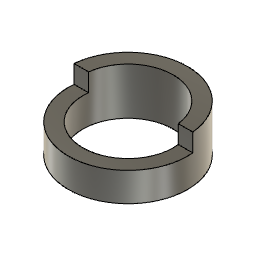
DISP_Ring_V2 v1 (Autodesk Fusion 360 design; units mm, degrees)
Autodesk Fusion 360 part; units mm, degrees
note: some values were not read from the file. Set by a fixed rule: which sketch regions a step uses.
sketch "Sketch1" plane through (0, 0, 0) normal (0, 0, 1) x (1, 0, 0)
  circle A0 centre (0, 0) radius 16.5
  circle A1 centre (0, 0) radius 12.5
  dimension "d1" = 33
  dimension "d2" = 25
  constraint coincident A0.centre A1.centre
  measures "d1" diameter of A0
  measures "d2" diameter of A1
extrude "Extrude1" add sketch "Sketch1" along normal blind 8
sketch "Sketch2" plane through (0, 0, 8) normal (0, 0, 1) x (-1, 0, 0)
  circle A0 centre (0, 0) radius 12.5
  circle A1 centre (0, 0) radius 16.5
  line L0 (-0.0363, -16.5) -> (-0.0363, -1.5) construction
  line L1 (-0.0363, -1.5) -> (16.4317, -1.5) construction
  line L2 (16.4317, -1.5) -> (-16.4317, -1.5)
  line L3 (-16.4317, -1.5) -> (-13.3757, -8.3419)
  dimension "d5" = 15
  dimension "d6" = 7.4934
  constraint coincident A1 L0.start
  constraint vertical L0
  constraint coincident A1 L1.end
  constraint perpendicular L0 L1
  constraint coincident A1 L2.end
  constraint parallel L1 L2
  measures "d5" distance of L0.start L0.end
  measures "d6" distance of L2.end L3.end
extrude "Extrude2" add sketch "Sketch2" along normal blind 5 contours A0 A1 L2 picked at (14.9574, -2.302)
